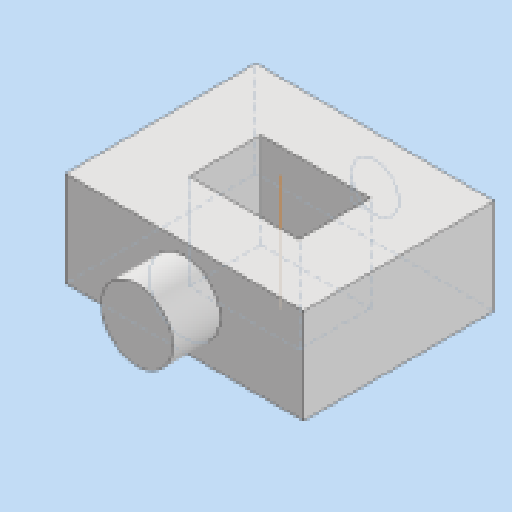
# Autodesk Inventor part: Pen_nib_stopper
Saved by Autodesk Inventor 2024 (Build 280153000, 153)
## iProperties
Created: 2025-02-15
Part Number: Pen_nib_stopper
Material: Generic
Document SubType Name: Modeling
Designer: XxPan
Density: 1 g/cm^3
Appearance: Default
Author: XxPan
Autodesk Inventor part; units mm, degrees
ref_plane "YZ Plane" through (0, 0, 0) normal (1, 0, 0) x (0, 1, 0)
ref_plane "XZ Plane" through (0, 0, 0) normal (0, 1, 0) x (-1, 0, 0)
ref_plane "XY Plane" through (0, 0, 0) normal (0, 0, 1) x (1, 0, 0)
sketch "Sketch1" plane through (0, 0, 0) normal (0, 1, 0) x (-1, 0, 0)
  line L0 (2.3, 1.5) -> (-2.3, 1.5)
  line L1 (-2.3, 1.5) -> (-2.3, -1.5)
  line L2 (-2.3, -1.5) -> (2.3, -1.5)
  line L3 (2.3, -1.5) -> (2.3, 1.5)
  line L4 (7, 0) -> (-7, 0) construction
  line L5 (0, -5.6) -> (0, 5.6) construction
  line L6 (5, 4) -> (-5, 4)
  line L7 (-5, 4) -> (-5, -4)
  line L8 (-5, -4) -> (5, -4)
  line L9 (5, -4) -> (5, 4)
  point P0 (0, 0)
  point P1 (2.3, 0)
  point P2 (0, 1.5)
  dimension "d1" = 4.6
  dimension "d2" = 3
  dimension "d3" = 10
  dimension "d16" = 2.5
  dimension "d17" = 2.5
  constraints: 16 end point, 4 parallel, 2 horizontal, 2 midpoint, 2 perpendicular, 2 point on line, 1 other
  measures "d1" distance of L2.end L1.end
  measures "d2" distance of L1.end L0.end
  measures "d3" distance of L8.end L7.end
  measures "d16" distance between parallel lines of L0 L6
  measures "d17" distance between parallel lines of L2 L8
extrude "Extrusion1" add sketch "Sketch1" along normal blind 4
sketch "Sketch2" plane through (-5, 0, 4) normal (0, 0, 1) x (1, 0, 0)
  circle A0 centre (5, 2) radius 1.5
  line L0 (0, 4) -> (10, 4) construction
  line L1 (5, -0.8) -> (5, 4.8) construction
  line L2 (0, 0) -> (0, 4) projected
  point P0 (5, 0)
  point P1 (0, 2)
  dimension "d7" = 3
  constraints: 2 midpoint, 1 centre point, 1 horizontal alignment
  measures "d7" diameter of A0
extrude "Extrusion2" add sketch "Sketch2" along normal blind 5
sketch "Sketch4" plane through (5, 0, -4) normal (0, 0, -1) x (-1, 0, 0)
  circle A0 centre (5, 1.8) radius 0.2 construction
  circle A1 centre (5, 1.8) radius 0.5
  line L0 (4.6464, 2.1536) -> (5, 2.5071)
  line L1 (5, 2.5071) -> (5.3536, 2.1536)
  point P0 (5, 0)
  dimension "d18" = 1
  constraints: 4 end point, 2 point on circle, 2 tangent, 1 centre point, 1 coincident, 1 perpendicular, 1 vertical alignment
  measures "d18" diameter of A1
extrude "Extrusion4" cut sketch "Sketch4" against normal blind 1
chamfer "Chamfer2" distance 0.2 angle 45 3 edges at (-0.1768, 2.3303, -4) (0, 1.3, -4) (0.1768, 2.3303, -4)
body "Solid1"
